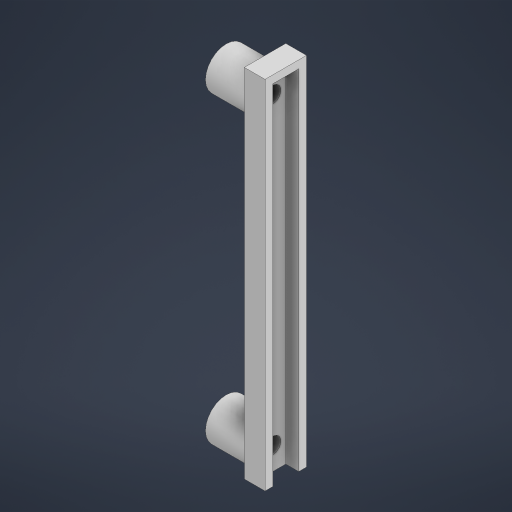
# Autodesk Inventor part: hs_intake_joint
Saved by Autodesk Inventor 2024 (Build 280153000, 153)
## iProperties
Created: 2023-10-10
Part Number: hs_intake_joint
Material: Generic
Document SubType Name: Modeling
Designer: Averey Ku
Density: 1 g/cm^3
Appearance: Default
Author: Averey Ku
Autodesk Inventor part; units mm, degrees
ref_plane "YZ Plane" through (0, 0, 0) normal (1, 0, 0) x (0, 1, 0)
ref_plane "XZ Plane" through (0, 0, 0) normal (0, 1, 0) x (-1, 0, 0)
ref_plane "XY Plane" through (0, 0, 0) normal (0, 0, 1) x (1, 0, 0)
sketch "Sketch1" plane through (0, 0, 0) normal (0, 1, 0) x (-1, 0, 0)
  line L0 (0, 3.1877) -> (3.1877, 3.1877)
  line L1 (3.1877, 3.1877) -> (3.1877, -3.175)
  line L2 (3.1877, -3.175) -> (0, -3.175)
  line L3 (0, 5.08) -> (5.08, 5.08)
  line L4 (5.08, 5.08) -> (5.08, -5.08)
  line L5 (5.08, -5.08) -> (0, -5.08)
  line L6 (0, -5.08) -> (0, -3.175)
  line L7 (0, 3.1877) -> (0, 5.08)
  point P0 (0, 0)
  dimension "d0" = 3.1877
  dimension "d1" = 5.08
  dimension "d2" = 10.16
  constraints: 16 end point, 4 parallel, 2 horizontal, 2 perpendicular
  measures "d0" distance of L1.end L2.end
  measures "d1" distance of L4.end L5.end
  measures "d2" distance of L3.end L4.end
extrude "Extrusion1" add sketch "Sketch1" along normal blind 85.4964
sketch "Sketch2" plane through (0, 85.4964, 0) normal (0, 1, 0) x (1, 0, 0)
  line L0 (0, -5.08) -> (0, -3.1877) projected
  line L1 (0, 5.08) -> (-5.08, 5.08) projected
  line L2 (0, -5.08) -> (-5.08, -5.08)
  line L3 (-5.08, -5.08) -> (-5.08, 5.08)
  line L4 (-5.08, 5.08) -> (0, 5.08)
  line L5 (0, 5.08) -> (0, -5.08)
  point P0 (0, 0)
  constraints: 8 end point, 2 parallel, 1 horizontal, 1 perpendicular
extrude "Extrusion2" add sketch "Sketch2" along normal blind 1.8923
sketch "Sketch3" plane through (-5.08, 0, -5.08) normal (-1, 0, 0) x (0, 0, 1)
  circle A0 centre (5.08, 5.4991) radius 1.9844
  circle A1 centre (5.08, 79.9973) radius 1.9844
  point P0 (5.08, 0)
  dimension "d7" = 3.9688
  dimension "d8" = 3.9688
  constraints: 2 centre point
  measures "d7" diameter of A0
  measures "d8" diameter of A1
extrude "Extrusion3" cut sketch "Sketch3" against normal blind 1.8923
sketch "Sketch4" plane through (-5.08, 5.4991, 0) normal (-1, 0, 0) x (0, 0, 1)
  circle A0 centre (0, 0) radius 1.9844 projected
  circle A1 centre (0, 0) radius 1.9844
  circle A2 centre (0, 0) radius 5.08
  line L0 (5.08, -5.4991) -> (5.08, 81.8896) projected
  circle A3 centre (0, 74.4982) radius 1.9844 projected
  circle A4 centre (0, 74.4982) radius 1.9844
  circle A5 centre (0, 74.4982) radius 5.08
  point P0 (0, -5.4991)
  constraints: 4 centre point, 4 coincident, 2 tangent, 1 concentric
extrude "Extrusion4" add sketch "Sketch4" along normal blind 9.525
body "Solid1"
